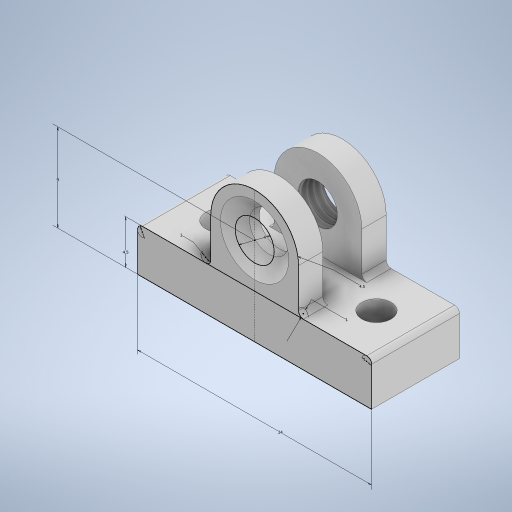
# Autodesk Inventor part: Hudson 1-72
Saved by Autodesk Inventor 2024.2 (Build 282272000, 272)
## iProperties
Created: 2024-11-02
Part Number: Hudson 1-72
Material: Genérico
Document SubType Name: Modeling
Designer: Monica Mora
Density: 1 g/cm^3
Appearance: Valor por defecto
Author: Monica Mora
Autodesk Inventor part; units mm, degrees
ref_plane "YZ Plane" through (0, 0, 0) normal (1, 0, 0) x (0, 1, 0)
ref_plane "XY Plane" through (0, 0, 0) normal (0, 0, 1) x (1, 0, 0)
sketch "Boceto1" plane through (0, 0, 0) normal (0, 0, 1) x (1, 0, 0)
  line L0 (0, 0) -> (-24, 0)
  line L1 (-24, 0) -> (-24, 4)
  line L2 (-23.5, 4.5) -> (-0.5, 4.5)
  line L3 (0, 4) -> (0, 0)
  arc A0 (-23.5, 4.5) -> (-24, 4) centre (-23.5, 4) ccw
  arc A1 (0, 4) -> (-0.5, 4.5) centre (-0.5, 4) ccw
  line L4 (-12, 0) -> (-12, 13.5) construction
  circle A2 centre (-12, 9) radius 2
  arc A3 (-7.5, 9) -> (-16.5, 9) centre (-12, 9) ccw
  line L5 (-16.5, 9) -> (-16.5, 5)
  line L6 (-7.5, 9) -> (-7.5, 5)
  arc A4 (-17, 4.5) -> (-16.5, 5) centre (-17, 5) ccw
  arc A5 (-7.5, 5) -> (-7, 4.5) centre (-7, 5) ccw
  dimension "d0" = 24
  dimension "d2" = 1
  dimension "d3" = 1
  dimension "d4" = 4.5
  dimension "d5" = 4.5
  dimension "d6" = 4
  dimension "d7" = 9
  dimension "d8" = 1
  dimension "d9" = 1
  constraints: 14 end point, 11 point on circle, 10 tangent, 6 centre point, 3 point on line, 2 parallel, 2 perpendicular, 2 vertical, 1 coincident, 1 horizontal, 1 midpoint
  measures "d0" distance of L0.start L0.end
  measures "d2" diameter of A0
  measures "d3" diameter of A1
  measures "d4" distance between parallel lines of L0 L2
  measures "d5" radius of A3
  measures "d6" diameter of A2
  measures "d7" distance from line of L0 A2.centre
  measures "d8" diameter of A5
  measures "d9" diameter of A4
extrude "Extrusión1" add sketch "Boceto1" against normal blind 9 contours L0 L1 A0 L2 A1 L3 | L2 A4 L5 A3 L6 A5 | A2
ref_plane "Plano de trabajo1" through (0, 13.5, 0) normal (0, 1, 0) x (-1, 0, 0)
sketch "Boceto2" plane through (0, 13.5, 0) normal (0, 1, 0) x (-1, 0, 0)
  line L0 (24, 0) -> (24, -9) projected
  line L1 (24, -4.5) -> (0, -4.5) construction
  line L2 (0, 0) -> (0, -9) projected
  line L3 (7.5, -9) -> (16.5, -9) projected
  line L4 (12, -9) -> (12, 0) construction
  line L5 (24, -6.5) -> (0, -6.5)
  line L6 (0, -6.5) -> (0, -2.5)
  line L7 (0, -2.5) -> (24, -2.5)
  line L8 (24, -2.5) -> (24, -6.5)
  circle A0 centre (20, -4.5) radius 1.5
  circle A1 centre (4, -4.5) radius 1.5
  point P0 (0, -4.5)
  point P1 (12, -6.5)
  point P2 (0, -6.5)
  dimension "d13" = 2
  dimension "d14" = 8
  dimension "d15" = 8
  dimension "d16" = 3
  dimension "d17" = 3
  constraints: 12 end point, 6 point on line, 5 midpoint, 2 centre point, 2 parallel, 1 horizontal, 1 perpendicular, 1 vertical
  measures "d13" distance between parallel lines of L1 L5
  measures "d14" distance from line of L4 A0.centre
  measures "d15" distance from line of L4 A1.centre
  measures "d16" diameter of A0
  measures "d17" diameter of A1
extrude "Extrusión2" cut sketch "Boceto2" against normal blind 9
hole "Agujero1" at (-20, 13.5, -4.5) at (-4, 13.5, -4.5) direction (0, -1, 0) diameter 3 end through all
hole "Agujero2" at (-12, 9, 0) direction (0, 0, -1) diameter 4 end through all countersink diameter 7 countersink angle 90
thread "Rosca1" size "M4x0.7" class "6H" standard "ANSI Metric M Profile" full length
equation "\"d15\" = d14"
